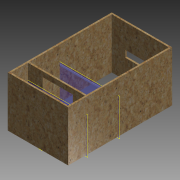
# Autodesk Inventor part: Spanplatten Gehäuse
Saved by Autodesk Inventor 2013 (Build 170138000, 138)
## iProperties
Created: 2012-07-26
Part Number: Spanplatten Gehäuse
Material: Edelstahl, 440C
Document SubType Name: Modeling
Designer: fivef
Density: 7.75 g/cm^3
Mass: 50743.6 g
Surface Area: 13924.8 cm^2
Volume: 6547.56 cm^3
Author: fivef
Autodesk Inventor part; units mm, degrees
ref_plane "YZ Plane" through (0, 0, 0) normal (1, 0, 0) x (0, 1, 0)
ref_plane "XZ Plane" through (0, 0, 0) normal (0, 1, 0) x (-1, 0, 0)
ref_plane "XY Plane" through (0, 0, 0) normal (0, 0, 1) x (1, 0, 0)
sketch "Skizze2" plane through (0, 0, 0) normal (0, 1, 0) x (-1, 0, 0)
  line L0 (-360, 300) -> (0, 300)
  line L1 (0, 300) -> (0, 0)
  line L2 (0, 0) -> (-360, 0)
  line L3 (-360, 0) -> (-360, 300)
  line L4 (-360, 300) -> (0, 0) construction
  line L5 (0, 300) -> (-360, 0) construction
  point P0 (-180, 150)
  dimension "d6" = 360
  dimension "d7" = 300
  constraints: 12 end point, 2 midpoint, 2 parallel, 1 horizontal, 1 perpendicular
  measures "d6" distance of L1.end L2.end
  measures "d7" distance of L0.end L1.end
extrude "Deckel oben" add sketch "Skizze2" along normal blind 10
hole "Bohrung1" at (5, 10, 50) direction (0, -1, 0) diameter 3 depth 20 tip angle 118
hole "Bohrung2" at (5, 10, 250) direction (0, -1, 0) diameter 3 depth 20 tip angle 118
ref_plane "Arbeitsebene5" through (185, -600, 0) normal (0, -1, 0) x (1, 0, 0)
sketch "Skizze8" plane through (185, -600, 0) normal (0, -1, 0) x (1, 0, 0)
  line L0 (-185, 300) -> (175, 300)
  line L1 (175, 300) -> (175, 0)
  line L2 (175, 0) -> (-185, 0)
  line L3 (-185, 0) -> (-185, 300)
  line L4 (-185, 300) -> (175, 0) construction
  line L5 (175, 300) -> (-185, 0) construction
  point P0 (-5, 150)
  dimension "d30" = 360
  dimension "d31" = 300
  constraints: 12 end point, 2 midpoint, 2 parallel, 1 horizontal, 1 perpendicular
  measures "d30" distance of L1.end L2.end
  measures "d31" distance of L0.end L1.end
extrude "Boden" add sketch "Skizze8" along normal blind 10 separate body
sketch "Skizze9" plane through (360, 305, 300) normal (1, 0, 0) x (0, 0, -1)
  line L0 (0, -305) -> (300, -305)
  line L1 (300, -305) -> (300, -905)
  line L2 (300, -905) -> (0, -905)
  line L3 (0, -905) -> (0, -305)
  point P0 (300, -305)
  dimension "d35" = 600
  dimension "d60" = 300
  dimension "d63" = 0
  constraints: 8 end point, 2 parallel, 1 horizontal, 1 perpendicular
  measures "d35" distance of L0.end L1.end
  measures "d60" distance of L0.start L0.end
  measures "d63" distance from line of point (300, -305) L1
extrude "Linke Wand" add sketch "Skizze9" against normal blind 10 separate body
ref_plane "Arbeitsebene4" through (185, -500, 0) normal (0, 1, 0) x (1, 0, 0)
sketch "Skizze10" plane through (190, -500, 100) normal (0, 1, 0) x (1, 0, 0)
  line L0 (-179.5454, 100) -> (160.4546, 100)
  line L1 (160.4546, 100) -> (160.4546, -200)
  line L2 (160.4546, -200) -> (-179.5454, -200)
  line L3 (-179.5454, -200) -> (-179.5454, 100)
  line L4 (-179.5454, 100) -> (160.4546, -200) construction
  line L5 (160.4546, 100) -> (-179.5454, -200) construction
  line L6 (-190, 100) -> (170, 100) projected
  point P0 (-9.5454, -50)
  dimension "d40" = 340
  dimension "d41" = 300
  dimension "d65" = 0
  constraints: 12 end point, 2 midpoint, 2 parallel, 1 horizontal, 1 perpendicular
  measures "d40" distance of L1.end L2.end
  measures "d41" distance of L0.end L1.end
  measures "d65" distance between parallel lines of L0 L6
extrude "Zwischenboden" add sketch "Skizze10" along normal blind 10 separate body
sketch "Skizze11" plane through (0, 610, 0) normal (-1, 0, 0) x (0, 0, 1)
  line L0 (0, -610) -> (300, -610)
  line L1 (300, -610) -> (300, -1210)
  line L2 (300, -1210) -> (0, -1210)
  line L3 (0, -1210) -> (0, -610)
  point P0 (300, -610)
  dimension "d45" = 600
  dimension "d61" = 300
  dimension "d64" = 0
  constraints: 8 end point, 2 parallel, 1 horizontal, 1 perpendicular
  measures "d45" distance of L0.end L1.end
  measures "d61" distance of L0.start L0.end
  measures "d64" distance from line of point (300, -610) L1
extrude "Rechte Wand" add sketch "Skizze11" against normal blind 10 bodies 1
sketch "Skizze15" plane through (190, -490, 100) normal (0, 1, 0) x (1, 0, 0)
  line L0 (-92.1258, -80) -> (87.8742, -80)
  line L1 (87.8742, -80) -> (87.8742, -170)
  line L2 (87.8742, -170) -> (-92.1258, -170)
  line L3 (-92.1258, -170) -> (-92.1258, -80)
  line L4 (-92.1258, -80) -> (87.8742, -170) construction
  line L5 (87.8742, -80) -> (-92.1258, -170) construction
  circle A0 centre (-185, -150) radius 1.5 projected
  circle A1 centre (-185, 50) radius 1.5 projected
  line L6 (-190, -200) -> (170, -200) projected
  line L7 (170, -200) -> (170, 100) projected
  line L8 (170, 100) -> (-190, 100) projected
  line L9 (-190, 100) -> (-190, -200) projected
  line L10 (170, 100) -> (-190, 100) projected
  line L11 (170, -200) -> (170, 100) projected
  point P0 (-2.1258, -125)
  dimension "d57" = 180
  dimension "d59" = 90
  dimension "d62" = 30
  constraints: 12 end point, 2 midpoint, 2 parallel, 1 horizontal, 1 perpendicular
  measures "d57" distance of L0.start L0.end
  measures "d59" distance of L0.end L1.end
  measures "d62" distance between parallel lines of L6 L2
extrude "Abtropfgitter" cut sketch "Skizze15" against normal blind 20 contours L0 L1 L2 L3 bodies 4
sketch "Skizze16" plane through (0, 10, 0) normal (0, 1, 0) x (1, 0, 0)
  line L0 (50.5996, -54.7496) -> (230.5977, -55.5818) projected
  line L1 (230.5289, -70.4701) -> (50.5308, -69.6379) projected
  line L2 (90, -116.3949) -> (270, -116.3949)
  line L3 (270, -116.3949) -> (270, -156.3949)
  line L4 (270, -156.3949) -> (90, -156.3949)
  line L5 (90, -156.3949) -> (90, -116.3949)
  dimension "d71" = 40
  dimension "d72" = 180
  constraints: 8 end point, 2 parallel, 1 horizontal, 1 perpendicular
  measures "d71" distance of L2.end L3.end
  measures "d72" distance of L3.end L4.end
extrude "öffnung oben" cut sketch "Skizze16" against normal blind 50 bodies 1
ref_plane "Arbeitsebene7" through (180, -250.9808, 190.5) normal (0, 1, 0) x (1, 0, 0)
sketch "Skizze17" plane through (180, -250.9808, 190.5) normal (0, 1, 0) x (1, 0, 0)
  line L0 (-25.2697, 55.6344) -> (-54.2694, 55.7685) projected
  line L1 (-169.5454, 190.5) -> (-169.5454, -109.5) projected
  line L2 (170.4546, -109.5) -> (170.4546, 190.5) projected
  line L3 (-169.5454, 0.5) -> (170.4546, 0.5)
  line L4 (170.4546, 0.5) -> (170.4546, -4.5)
  line L5 (170.4546, -4.5) -> (-169.5454, -4.5)
  line L6 (-169.5454, -4.5) -> (-169.5454, 0.5)
  point P0 (-180, 190.5)
  dimension "d75" = 5
  dimension "d76" = 340
  constraints: 8 end point, 2 parallel, 1 horizontal, 1 perpendicular
  measures "d75" distance of L5.end L3.start
  measures "d76" distance of L3.start L3.end
extrude "ventilhalter stange" add sketch "Skizze17" against normal blind 1 bodies 4
